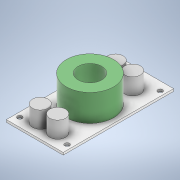
# Autodesk Inventor part: a1401220
Saved by Autodesk Inventor 2020 (Build 240168000, 168)
## iProperties
Created: 2024-02-05
Part Number: a1401220
Material: Типовые
Document SubType Name: Modeling
Designer: 4s
Density: 1 g/cm^3
Appearance: По умолчанию
Author: 4s
Autodesk Inventor part; units mm, degrees
ref_plane "YZ Plane" through (0, 0, 0) normal (1, 0, 0) x (0, 1, 0)
ref_plane "XZ Plane" through (0, 0, 0) normal (0, 1, 0) x (-1, 0, 0)
ref_plane "XY Plane" through (0, 0, 0) normal (0, 0, 1) x (1, 0, 0)
sketch "Эскиз1" plane through (0, 0, 0) normal (0, 1, 0) x (-1, 0, 0)
  line L0 (18, -35) -> (-18, -35)
  line L1 (-18, -35) -> (-18, 35)
  line L2 (-18, 35) -> (18, 35)
  line L3 (18, 35) -> (18, -35)
  line L4 (18, -35) -> (-18, 35) construction
  line L5 (-18, -35) -> (18, 35) construction
  line L6 (15, -29.5) -> (-15, -29.5) construction
  line L7 (-15, -29.5) -> (-15, 29.5) construction
  line L8 (-15, 29.5) -> (15, 29.5) construction
  line L9 (15, 29.5) -> (15, -29.5) construction
  line L10 (15, -29.5) -> (-15, 29.5) construction
  line L11 (-15, -29.5) -> (15, 29.5) construction
  circle A0 centre (15, -29.5) radius 1.5
  line L12 (0, 0) -> (0, -35) construction
  line L13 (18, 0) -> (-18, 0) construction
  line L14 (15, -29.5) -> (-15, 29.5) construction
  circle A1 centre (-15, -29.5) radius 1.5
  line L15 (-18, 0) -> (18, 0) construction
  circle A2 centre (15, 29.5) radius 1.5
  circle A3 centre (-15, 29.5) radius 1.5
  point P0 (0, 0)
  dimension "d0" = 36
  dimension "d1" = 70
  dimension "d2" = 30
  dimension "d3" = 59
  dimension "d4" = 3
  constraints: 32 end point, 9 midpoint, 5 symmetric about line, 4 centre point, 4 parallel, 2 horizontal, 2 perpendicular, 1 coincident, 3 other
  measures "d0" distance of L0.start L0.end
  measures "d1" distance of L0.end L1.end
  measures "d2" distance of L6.start L6.end
  measures "d3" distance of L6.end L7.end
  measures "d4" diameter of A0
extrude "Выдавливание1" add sketch "Эскиз1" along normal blind 1.5
sketch "Эскиз2" plane through (0, 1.5, 0) normal (0, 1, 0) x (1, 0, 0)
  circle A0 centre (0, 0) radius 15
  circle A1 centre (0, 0) radius 7.5
  dimension "d7" = 30
  dimension "d8" = 15
  constraints: 2 centre point, 2 coincident
  measures "d7" diameter of A0
  measures "d8" diameter of A1
extrude "Выдавливание2" add sketch "Эскиз2" along normal blind 17
sketch "Эскиз4" plane through (0, 1.5, 0) normal (0, 1, 0) x (1, 0, 0)
  circle A0 centre (-5.5, -26) radius 5
  line L0 (-18, -35) -> (18, -35) projected
  circle A1 centre (5.5, -26) radius 5
  line L1 (-18, 35) -> (-18, -35) projected
  line L2 (-18, 35) -> (-18, -35) construction
  line L3 (-18, 0) -> (18, 0) construction
  line L4 (18, -35) -> (18, 35) construction
  circle A2 centre (-5.5, 21.5) radius 5
  circle A3 centre (5.5, 21.5) radius 5
  line L5 (18, 35) -> (-18, 35) projected
  point P0 (0, 0)
  dimension "d11" = 10
  dimension "d12" = 9
  dimension "d13" = 10
  dimension "d14" = 9
  dimension "d15" = 11
  dimension "d16" = 12.5
  dimension "d19" = 10
  dimension "d20" = 10
  dimension "d21" = 13.5
  dimension "d22" = 13.5
  dimension "d23" = 11
  dimension "d24" = 12.5
  constraints: 4 centre point, 2 end point, 2 midpoint
  measures "d11" diameter of A0
  measures "d12" distance from line of L0 A0.centre
  measures "d13" diameter of A1
  measures "d14" distance from line of L0 A1.centre
  measures "d15" distance of A0.centre A1.centre
  measures "d16" distance from line of L1 A0.centre
  measures "d19" diameter of A2
  measures "d20" diameter of A3
  measures "d21" distance from line of L5 A2.centre
  measures "d22" distance from line of L5 A3.centre
  measures "d23" distance of A3.centre A2.centre
  measures "d24" distance from line of L1 A2.centre
extrude "Выдавливание3" add sketch "Эскиз4" along normal blind 10.5
ref_plane "РабПлоскость1" through (-18, 0, 0) normal (0, 0, 1) x (1, 0, 0)
